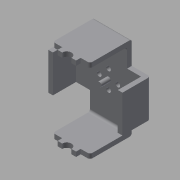
# Autodesk Inventor part: ShoulderPlateXZ
Saved by Autodesk Inventor 2017 (Build 210142000, 142)
## iProperties
Created: 2017-05-07
Part Number: ShoulderPlateXZ
Material: Generic
Document SubType Name: Modeling
Designer: zallen
Density: 1 g/cm^3
Appearance: Default
Author: zallen
Autodesk Inventor part; units mm, degrees
ref_plane "YZ Plane" through (0, 0, 0) normal (1, 0, 0) x (0, 1, 0)
ref_plane "XZ Plane" through (0, 0, 0) normal (0, 1, 0) x (-1, 0, 0)
ref_plane "XY Plane" through (0, 0, 0) normal (0, 0, 1) x (1, 0, 0)
sketch "Sketch1" plane through (0, 0, 0) normal (0, 0, 1) x (1, 0, 0)
  circle A0 centre (0, -12.7) radius 3.175
  circle A1 centre (12.7, 0) radius 3.175
  circle A2 centre (0, 12.7) radius 3.175
  circle A3 centre (-12.7, 0) radius 3.175
  line L0 (25.4, 57.15) -> (-25.4, 57.15)
  line L1 (-25.4, 57.15) -> (-25.4, -57.15)
  line L2 (-25.4, -57.15) -> (25.4, -57.15)
  line L3 (25.4, -57.15) -> (25.4, 57.15)
  point P0 (0, 0)
  dimension "d1" = 6.35
  dimension "d2" = 12.7
  dimension "d5" = 360
  dimension "d13" = 25.4
  dimension "d14" = 57.15
  dimension "d15" = 57.15
  dimension "d16" = 25.4
  constraints: 8 end point, 4 centre point, 2 parallel, 1 horizontal, 1 perpendicular, 9 other
  measures "d1" diameter of A0
  measures "d2" distance of point (0, 0) A0.centre
  measures "d13" distance from line of point (0, 0) L1
  measures "d14" distance from line of point (0, 0) L2
  measures "d15" distance from line of L0 point (0, 0)
  measures "d16" distance from line of L3 point (0, 0)
extrude "Extrusion3" add sketch "Sketch1" along normal blind 6.35
sketch "Sketch3" plane through (0, 0, 6.35) normal (0, 0, 1) x (1, 0, 0)
  line L0 (25.4, 57.15) -> (-25.4, 57.15) projected
  line L1 (25.4, 57.15) -> (25.4, 50.8)
  line L2 (25.4, -57.15) -> (25.4, 57.15) projected
  line L3 (25.4, 50.8) -> (-25.4, 50.8)
  line L4 (-25.4, 57.15) -> (-25.4, -57.15) projected
  line L5 (-25.4, 57.15) -> (25.4, 57.15)
  line L6 (-25.4, -57.15) -> (25.4, -57.15) projected
  line L7 (25.4, -57.15) -> (25.4, -50.8)
  line L8 (25.4, -50.8) -> (-25.4, -50.8)
  line L9 (-25.4, -50.8) -> (-25.4, -57.15)
  line L10 (-25.4, -57.15) -> (25.4, -57.15)
  point P0 (0, 0)
  dimension "d19" = 6.35
  dimension "d20" = 6.35
  constraints: 14 end point, 5 perpendicular, 3 point on line
  measures "d19" distance of L0.start L1.end
  measures "d20" distance of L2.start L7.end
extrude "Extrusion4" add sketch "Sketch3" along normal blind 50.8 contours L1 L3 L4 L0 | L2 L6 L4 L8
fillet "Fillet1" radius 3.175 8 edges at (25.4, 53.975, 57.15) (25.4, -53.975, 57.15) (-25.4, -53.975, 57.15) (-25.4, 53.975, 57.15) (0, -57.15, 0) (0, 57.15, 0) (0, -50.8, 6.35) (0, 50.8, 6.35)
sketch "Sketch6" plane through (0, 0, 6.35) normal (0, 0, 1) x (1, 0, 0)
  circle A0 centre (0, 0) radius 3.175
  dimension "d50" = 6.35
  constraints: 1 centre point, 1 coincident
  measures "d50" diameter of A0
extrude "Extrusion6" add sketch "Sketch6" along normal blind 12.7
sketch "Sketch7" plane through (-25.4, 57.15, 3.175) normal (0, 1, 0) x (1, 0, 0)
  line L0 (47.625, -53.975) -> (3.175, -53.975) projected
  line L1 (0, 0) -> (0, -50.8) projected
  line L2 (47.625, -53.975) -> (3.175, -53.975) projected
  line L3 (38.1, -53.975) -> (38.1, -60.325)
  line L4 (12.7, -60.325) -> (12.7, -53.975)
  line L5 (38.1, -60.325) -> (31.75, -60.325)
  line L6 (19.05, -60.325) -> (12.7, -60.325)
  line L7 (38.1, -53.975) -> (12.7, -53.975)
  arc A0 (31.75, -60.325) -> (25.4, -53.975) centre (25.4, -60.325) ccw
  arc A1 (25.4, -53.975) -> (19.05, -60.325) centre (25.4, -60.325) ccw
  point P0 (25.4, 3.175)
  dimension "d57" = 38.1
  dimension "d58" = 12.7
  dimension "d59" = 6.35
  dimension "d60" = 6.35
  dimension "d66" = 6.35
  dimension "d67" = 25.4
  dimension "d68" = 6.35
  dimension "d69" = 25.4
  constraints: 10 end point, 4 point on circle, 2 centre point, 2 collinear, 2 perpendicular, 2 point on line, 1 horizontal, 1 midpoint
  measures "d57" distance between parallel lines of L1 L3
  measures "d58" distance between parallel lines of L1 L4
  measures "d59" distance between parallel lines of L0 L5
  measures "d60" distance between parallel lines of L0 L6
  measures "d66" distance from line of L0 A0.centre
  measures "d67" distance from line of L1 A0.centre
  measures "d68" distance from line of L0 A1.centre
  measures "d69" distance from line of L1 A1.centre
extrude "Extrusion7" add sketch "Sketch7" against normal blind 6.35
sketch "Sketch8" plane through (-25.4, -57.15, 3.175) normal (0, -1, 0) x (1, 0, 0)
  line L0 (12.7, 53.975) -> (12.7, 60.325) projected
  line L1 (12.7, 53.975) -> (12.7, 60.325)
  line L2 (38.1, 60.325) -> (38.1, 53.975) projected
  line L3 (38.1, 60.325) -> (38.1, 53.975)
  line L4 (38.1, 53.975) -> (25.4, 53.975)
  line L5 (47.625, 53.975) -> (3.175, 53.975) projected
  line L6 (12.7, 53.975) -> (25.4, 53.975)
  line L7 (12.7, 60.325) -> (19.05, 60.325) projected
  line L8 (12.7, 60.325) -> (19.05, 60.325)
  line L9 (31.75, 60.325) -> (38.1, 60.325) projected
  line L10 (38.1, 60.325) -> (31.75, 60.325)
  arc A0 (19.05, 60.325) -> (25.4, 53.975) centre (25.4, 60.325) ccw
  arc A1 (25.4, 53.975) -> (31.75, 60.325) centre (25.4, 60.325) ccw
  line L11 (0, 0) -> (0, 50.8) projected
  point P0 (25.4, -3.175)
  dimension "d72" = 6.35
  dimension "d73" = 6.35
  dimension "d74" = 25.4
  dimension "d75" = 25.4
  constraints: 12 end point, 4 collinear, 4 point on circle, 2 centre point, 2 midpoint, 1 horizontal, 1 point on line
  measures "d72" distance from line of L5 A0.centre
  measures "d73" distance from line of L4 A1.centre
  measures "d74" distance from line of L11 A0.centre
  measures "d75" distance from line of L11 A1.centre
extrude "Extrusion8" add sketch "Sketch8" against normal blind 6.35
sketch "Sketch9" plane through (0, 0, 6.35) normal (0, 0, 1) x (1, 0, 0)
  line L0 (-50.8, 25.4) -> (50.8, 25.4)
  line L1 (50.8, 25.4) -> (50.8, -25.4)
  line L2 (50.8, -25.4) -> (-50.8, -25.4)
  line L3 (-50.8, -25.4) -> (-50.8, 25.4)
  line L4 (-50.8, 25.4) -> (50.8, -25.4) construction
  line L5 (50.8, 25.4) -> (-50.8, -25.4) construction
  line L6 (25.4, -47.625) -> (25.4, 47.625) projected
  line L7 (25.4, 25.4) -> (25.4, -25.4)
  line L8 (-25.4, 53.975) -> (-25.4, -53.975) projected
  line L9 (-25.4, 25.4) -> (-25.4, -25.4)
  point P0 (0, 0)
  dimension "d78" = 101.6
  dimension "d79" = 50.8
  constraints: 16 end point, 8 point on line, 2 midpoint, 2 parallel, 1 horizontal, 1 perpendicular
  measures "d78" distance of L1.end L2.end
  measures "d79" distance of L0.end L1.end
extrude "Extrusion9" add sketch "Sketch9" against normal blind 6.35 contours L0 L8 L2 L3 | L0 L1 L2 L6
sketch "Sketch11" plane through (0, 0, 6.35) normal (0, 0, 1) x (1, 0, 0)
  line L0 (-25.4, -25.4) -> (-50.8, -25.4) projected
  line L1 (-50.8, -25.4) -> (-44.45, -25.4)
  line L2 (-44.45, -25.4) -> (-44.45, 25.4)
  line L3 (-25.4, 25.4) -> (-50.8, 25.4) projected
  line L4 (-50.8, -25.4) -> (-50.8, 25.4) projected
  line L5 (-50.8, 25.4) -> (-50.8, -25.4)
  line L6 (50.8, -25.4) -> (50.8, 25.4) projected
  line L7 (50.8, -25.4) -> (50.8, 25.4)
  line L8 (25.4, 25.4) -> (50.8, 25.4) projected
  line L9 (50.8, 25.4) -> (44.45, 25.4)
  line L10 (44.45, 25.4) -> (44.45, -25.4)
  line L11 (50.8, -25.4) -> (25.4, -25.4) projected
  line L12 (44.45, -25.4) -> (50.8, -25.4)
  point P0 (0, 0)
  dimension "d84" = 6.35
  dimension "d85" = 6.35
  constraints: 14 end point, 3 collinear, 3 point on line, 2 perpendicular
  measures "d84" distance of L0.end L1.end
  measures "d85" distance of L6.end L9.end
extrude "Extrusion11" add sketch "Sketch11" along normal blind 31.75
fillet "Fillet3" radius 3.175 2 edges at (50.8, 0, 0) (-50.8, 0, 0)
sketch "Sketch18" plane through (0, 0, 38.1) normal (0, 0, 1) x (1, 0, 0)
  line L0 (-50.8, 25.4) -> (-50.8, -25.4) projected
  line L1 (-50.8, -25.4) -> (50.8, -25.4)
  line L2 (50.8, -25.4) -> (50.8, 25.4)
  line L3 (50.8, 25.4) -> (-50.8, 25.4)
  line L4 (-50.8, 25.4) -> (-50.8, -25.4)
  circle A0 centre (-14.1478, -14.1478) radius 3.175
  circle A1 centre (14.1478, -14.1478) radius 3.175
  circle A2 centre (14.1478, 14.1478) radius 3.175
  circle A3 centre (-14.1478, 14.1478) radius 3.175
  circle A4 centre (0, 0) radius 3.175
  dimension "d132" = 6.35
  dimension "d137" = 360
  dimension "d139" = 6.35
  constraints: 8 end point, 5 centre point, 2 parallel, 1 coincident, 1 horizontal, 1 perpendicular, 9 other
  measures "d132" diameter of A0
  measures "d139" diameter of A4
extrude "Extrusion16" add sketch "Sketch18" along normal blind 6.35
body "Solid2"
